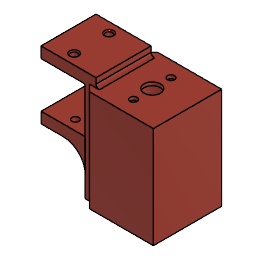
Base_motor_ (Autodesk Fusion 360 design; units mm, degrees)
Autodesk Fusion 360 part; units mm, degrees
sketch "Sketch1" plane through (0, 0, 0) normal (0, 0, 1) x (1, 0, 0)
  line L0 (0, 0) -> (25, 0)
  line L1 (25, 0) -> (25, 25)
  line L2 (25, 25) -> (0, 25)
  line L3 (0, 25) -> (0, 0)
  circle A0 centre (13, 12.5) radius 12.6
  line L4 (0, 25) -> (-5, 25)
  line L5 (-5, 25) -> (-5, 0)
  line L6 (-5, 0) -> (0, 0)
  line L7 (0, 0) -> (0, 25)
  line L8 (0, 25) -> (0, 28)
  line L9 (0, 28) -> (29, 28)
  line L10 (29, 28) -> (29, -3)
  line L11 (29, -3) -> (0, -3)
  line L12 (0, -3) -> (0, 28)
  dimension "d1" = 25
  dimension "d2" = 25
  dimension "d3" = 25.2
  dimension "d4" = 5
  dimension "d5" = 25
  dimension "d43" = 12.5
  dimension "d44" = 13
  dimension "d45" = 3
  constraint horizontal L0
  constraint vertical L1
  constraint horizontal L2
  constraint vertical L3
  constraint coincident L0.start L3.end
  constraint horizontal L4
  constraint vertical L5
  constraint horizontal L6
  constraint vertical L7
  constraint perpendicular L4 L8
  constraint horizontal L9
  constraint vertical L10
  constraint horizontal L11
  constraint vertical L12
  measures "d1" distance of L0.start L0.end
  measures "d2" distance of L0.start L2.end
  measures "d3" diameter of A0
  measures "d4" distance of L3 L5
  measures "d5" distance of L4 L6
  measures "d43" distance of L0 A0.centre
  measures "d44" distance of L3 A0.centre
  measures "d45" distance of L2.end L8.end
extrude "Extrude1" add sketch "Sketch1" along normal blind 70 contours L0 L2 L3 A0 L7 L12 | L3 L4 L5 L6 L7 L12 | L0 L1 L2 A0 L8 L9 L10 L11 L12 | L0 L1 A0 | L1 L2 A0 makes body 1
sketch "Sketch2" plane through (-5, 0, 0) normal (-1, 0, 0) x (0, -1, 0)
  line L0 (-25, 0) -> (0, 0)
  line L1 (0, 0) -> (0, 70)
  line L2 (0, 70) -> (-25, 70)
  line L3 (-25, 70) -> (-25, 0)
  line L4 (-12.5, 70) -> (-12.5, 60) construction
  circle A0 centre (-12.5, 60) radius 1.55
  line L5 (-25, 70) -> (0, 70)
  line L6 (0, 70) -> (0, 73)
  line L7 (0, 73) -> (-25, 73)
  line L8 (-25, 73) -> (-25, 70)
  dimension "d8" = 10
  dimension "d9" = 3.1
  dimension "d12" = 3
  dimension "d13" = 25
  constraint midpoint L2 L4.start
  constraint perpendicular L2 L4
  constraint coincident L4.end A0.centre
  constraint horizontal L5
  constraint vertical L6
  constraint horizontal L7
  constraint vertical L8
  constraint coincident L2.end L3.start
  measures "d8" distance of L4.start L4.end
  measures "d9" diameter of A0
  measures "d12" distance of L5 L7
  measures "d13" distance of L6 L8
extrude "Extrude2" cut sketch "Sketch2" against normal blind 6 contours A0 bodies 1
extrude "Extrude3" add sketch "Sketch2" along normal blind 20 separate body contours L2 L5 L6 L7 L8 makes body 2
sketch "Sketch3" plane through (0, 0, 73) normal (0, 0, 1) x (-1, 0, 0)
  line L0 (5, 0) -> (5, -25)
  line L1 (5, -25) -> (25, -25)
  line L2 (25, -25) -> (25, 0)
  line L3 (25, 0) -> (5, 0)
  circle A0 centre (14.5, -20.45) radius 1.55
  line L4 (25, -12.5) -> (5, -12.5) construction
  circle A1 centre (14.5, -4.55) radius 1.55
  dimension "d17" = 3.1
  dimension "d28" = 10.5
  constraint midpoint L2 L4.start
  constraint midpoint L0 L4.end
  constraint symmetric A0 L4 A1
  measures "d17" diameter of A0
  measures "d28" distance of L2 A0.centre
extrude "Extrude4" cut sketch "Sketch3" against normal blind 3 contours A0 | A1 bodies 2
extrude "Extrude5" add 1 faces at (-3.2, 12.5, 70) along direction (0, 0, 1) blind 3 on bodies 1 bodies 1 2
extrude "Extrude6" add 1 faces at (-8.8891, 12.5, 73) along direction (0, 0, 1) blind 2 on bodies 1 bodies 1
extrude "Extruir7" cut 1 faces at (-3.2, 12.5, 0) along direction (0, 0, 1) blind 15 on bodies 1 bodies 1
fillet "Empalme3" radius 0.5 1 edges at (-5, 12.5, 70) on bodies 1
ref_plane "PlanoDeObra1" through (0, 0, 49.3) normal (0, 0, 1) x (1, 0, 0)
sketch "Boceto4" plane through (0, 0, 49.3) normal (0, 0, 1) x (1, 0, 0)
  line L0 (-0.0315, 25) -> (-25, 25)
  line L1 (-25, 25) -> (-25, 0.0829)
  line L2 (-25, 0.0829) -> (-0.0315, 0.0829)
  line L3 (-0.0315, 0.0829) -> (-0.0315, 25)
  line L4 (-25, 25) -> (-14.5, 25)
  line L5 (-14.5, 25) -> (-14.5, 21.9)
  circle A0 centre (-14, 20.4329) radius 1.55
  line L6 (-0.0315, 12.5414) -> (-25, 12.5414) construction
  circle A1 centre (-14, 4.65) radius 1.55
  dimension "d34" = 10.5
  dimension "d35" = 3.1
  dimension "d36" = 3.1
  constraint horizontal L0
  constraint vertical L1
  constraint horizontal L2
  constraint vertical L3
  constraint perpendicular L1 L4
  constraint perpendicular L0 L5
  constraint coincident L5.end A0
  constraint midpoint L3 L6.start
  constraint midpoint L1 L6.end
  constraint symmetric A0 L6 A1
  measures "d34" distance of L0.end L4.end
  measures "d35" distance of L4.end L5.end
  measures "d36" diameter of A0
extrude "Extruir8" add sketch "Boceto4" against normal blind 5 bodies 1
fillet "Empalme4" radius 10 1 edges at (-5, 12.5414, 44.3) on bodies 1
fillet "Empalme5" radius 0.5 4 edges at (-15.4451, 4.0895, 44.3) (-15.4451, 19.8724, 44.3) (-13.0549, 3.9895, 75) (-13.0549, 19.8895, 75) on bodies 1
sketch "Sketch5" plane through (0, 0, 75) normal (0, 0, 1) x (-1, 0, 0)
  circle A0 centre (14.5, -4.55) radius 2.05
  circle A1 centre (-13, -12.5) radius 12.6
  line L0 (0, -25) -> (25, -25)
  line L1 (25, -25) -> (25, 0)
  line L2 (25, 0) -> (0, 0)
  line L3 (0, 0) -> (0, 3)
  line L4 (0, 3) -> (-29, 3)
  line L5 (-29, 3) -> (-29, -28)
  line L6 (-29, -28) -> (0, -28)
  line L7 (0, -28) -> (0, -25)
  circle A2 centre (14.5, -20.45) radius 2.05
  line L8 (0, -28) -> (-29, -28)
  line L9 (-29, -28) -> (-29, 3)
  line L10 (-29, 3) -> (0, 3)
  line L11 (0, 3) -> (0, -28)
  circle A3 centre (-13, -21) radius 1.6
  circle A4 centre (-13, -4) radius 1.6
  circle A5 centre (-13, -12.5) radius 3.7
  dimension "d50" = 3.2
  dimension "d51" = 3.2
  dimension "d58" = 7.4
  dimension "d59" = 8.5
  constraint horizontal L8
  constraint vertical L9
  constraint horizontal L10
  constraint vertical L11
  constraint coincident L4.end L5.start
  constraint coincident L6.end L7.start
  constraint concentric A1 A5
  measures "d50" diameter of A3
  measures "d51" diameter of A4
  measures "d58" diameter of A5
  measures "d59" distance of A4.centre A1.centre
extrude "Extrude9" add sketch "Sketch5" along normal blind 2 contours A1 | L3 L4 L5 L6 L7 L8 L9 L10 L11 bodies 1
extrude "Extrude10" cut 1 faces at (-3.2, 12.5, 15) along direction (0, 0, 1) blind 10 on bodies 1 bodies 1
extrude "Extruir13" cut sketch "Sketch5" against normal blind 4 contours A1 | L3 L4 L5 L6 L7 L8 L9 L10 L11 bodies 1
extrude "Extruir15" cut 1 faces at (24.9, 12.5, 77) along direction (0, 0, -1) blind 3 on bodies 1 bodies 1
extrude "Extruir16" add sketch "Sketch5" against normal blind 5.5 contours A1 bodies 1
extrude "Extruir17" cut sketch "Sketch5" against normal blind 4 contours A1 bodies 1
fillet "Empalme7" radius 1.5 1 edges at (0, 12.5, 71) on bodies 1
chamfer "Chaflán1" distance 3 angle 45 1 edges at (0, 0, 48) on bodies 1
chamfer "Chaflán1" distance 3 angle 45 1 edges at (0, 25, 48) on bodies 1
equation "d33 = 15 mm + 20.2 mm + 14.3 mm - 0.2 mm"
